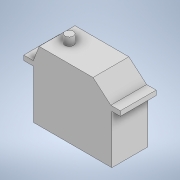
# Autodesk Inventor part: servospt35
Saved by Autodesk Inventor 2020 (Build 240168000, 168)
## iProperties
Created: 2021-03-17
Part Number: servospt35
Material: Generic
Document SubType Name: Modeling
Designer: super
Density: 1 g/cm^3
Appearance: Default
Author: super
Autodesk Inventor part; units mm, degrees
ref_plane "YZ Plane" through (0, 0, 0) normal (1, 0, 0) x (0, 1, 0)
ref_plane "XZ Plane" through (0, 0, 0) normal (0, 1, 0) x (-1, 0, 0)
ref_plane "XY Plane" through (0, 0, 0) normal (0, 0, 1) x (1, 0, 0)
sketch "Sketch1" plane through (0, 0, 0) normal (0, 0, 1) x (1, 0, 0)
  line L0 (0, 0) -> (65.7, 0)
  line L1 (65.7, 0) -> (65.7, 40.8)
  line L2 (0, 40.8) -> (0, 0)
  line L3 (0, 40.8) -> (-8, 40.8)
  line L4 (-8, 40.8) -> (-8, 44.8)
  line L5 (-8, 44.8) -> (0, 44.8)
  line L6 (0, 44.8) -> (4.8644, 57.5)
  line L7 (4.8644, 57.5) -> (49.9378, 57.5)
  line L8 (49.9378, 57.5) -> (64.8064, 44.8)
  line L9 (64.8064, 44.8) -> (72.8064, 44.8)
  line L10 (72.8064, 44.8) -> (72.8064, 40.8)
  line L11 (72.8064, 40.8) -> (65.7, 40.8)
  dimension "d0" = 65.7
  dimension "d1" = 40.8
  dimension "d2" = 4
  dimension "d9" = 57.5
  dimension "d13" = 8
  dimension "d14" = 8
  constraints: 24 end point, 3 horizontal, 2 parallel, 2 perpendicular, 2 point on line, 1 vertical
  measures "d0" distance of L2.start L1.end
  measures "d1" distance of L1.end L0.end
  measures "d2" distance of L3.end L4.end
  measures "d9" vertical distance of L0.start L6.end
  measures "d13" distance of L2.start L3.end
  measures "d14" distance of L8.end L9.end
extrude "Extrusion1" add sketch "Sketch1" against normal blind 30
sketch "Sketch2" plane through (4.8644, 57.5, 0) normal (0, 1, 0) x (1, 0, 0)
  circle A0 centre (10.1356, 15) radius 3.5
  line L0 (-12.8644, 30) -> (-4.8644, 30) projected
  point P0 (-4.8644, 0)
  dimension "d5" = 7
  dimension "d6" = 15
  dimension "d7" = 15
  constraints: 1 centre point
  measures "d5" diameter of A0
  measures "d6" distance from line of A0.centre L0
  measures "d7" horizontal distance of L0.end A0.centre
extrude "Extrusion2" add sketch "Sketch2" along normal blind 6.8
body "Solid1"
